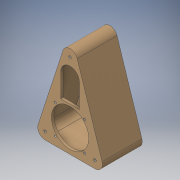
# Autodesk Inventor part: Nathan_New_LED_Speaker
Saved by Autodesk Inventor 2016 (Build 200138000, 138)
## iProperties
Created: 2018-09-25
Part Number: Nathan_New_LED_Speaker
Material: Generic
Document SubType Name: Modeling
Designer: Student
Density: 1 g/cm^3
Appearance: Default
Author: Student
Autodesk Inventor part; units mm, degrees
ref_plane "YZ Plane" through (0, 0, 0) normal (1, 0, 0) x (0, 1, 0)
ref_plane "XZ Plane" through (0, 0, 0) normal (0, 1, 0) x (-1, 0, 0)
ref_plane "XY Plane" through (0, 0, 0) normal (0, 0, 1) x (1, 0, 0)
sketch "Sketch1" plane through (0, 0, 0) normal (0, 0, 1) x (1, 0, 0)
  arc A0 (0.6195, 16.618) -> (12.7, 0) centre (12.7, 12.7) ccw
  arc A1 (63.5, 182.0332) -> (51.4195, 173.2512) centre (63.5, 169.3332) ccw
  line L0 (0.6195, 16.618) -> (51.4195, 173.2512)
  arc A2 (114.3, 0) -> (126.3805, 16.618) centre (114.3, 12.7) ccw
  arc A3 (75.5805, 173.2512) -> (63.5, 182.0332) centre (63.5, 169.3332) ccw
  line L1 (126.3805, 16.618) -> (75.5805, 173.2512)
  line L2 (12.7, 0) -> (114.3, 0)
  line L3 (63.5, 50.8) -> (63.5, 44.45)
  circle A4 centre (63.5, 44.45) radius 38.1
  circle A5 centre (33.655, 74.295) radius 2.1082
  circle A6 centre (93.345, 74.295) radius 2.1082
  circle A7 centre (93.345, 14.605) radius 2.1082
  circle A8 centre (33.655, 14.605) radius 2.1082
  line L4 (63.5, 82.55) -> (63.5, 86.36)
  line L5 (63.5, 86.36) -> (82.55, 86.36)
  line L6 (63.5, 86.36) -> (44.45, 86.36)
  line L7 (82.55, 86.36) -> (82.55, 134.62)
  line L8 (44.45, 86.36) -> (44.45, 134.62)
  arc A9 (82.55, 134.62) -> (44.45, 134.62) centre (63.5, 134.62) ccw
  point P0 (0, 0)
  dimension "d30" = 76.2
  dimension "d7" = 25.4
  dimension "d9" = 12.7
  dimension "d10" = 12.7
  dimension "d11" = 12.7
  dimension "d14" = 101.6
  dimension "d15" = 35.938
  dimension "d16" = 72.031
  dimension "d17" = 12.7
  dimension "d18" = 169.3332
  dimension "d19" = 109.3442
  dimension "d20" = 164.6651
  dimension "d21" = 164.6651
  dimension "d29" = 6.35
  dimension "d33" = 4.2164
  dimension "d34" = 4.2164
  dimension "d35" = 4.2164
  dimension "d36" = 4.2164
  dimension "d50" = 3.81
  dimension "d51" = 19.05
  dimension "d52" = 19.05
  dimension "d53" = 48.26
  dimension "d54" = 48.26
  constraints: 18 end point, 10 point on circle, 9 centre point, 4 vertical, 3 horizontal, 3 tangent, 1 coincident, 1 vertical alignment, 2 other
  measures "d7" diameter of A0
  measures "d9" radius of A2
  measures "d10" radius of A3
  measures "d11" radius of A1
  measures "d14" distance of L2.start L2.end
  measures "d15" angle of L1 L0
  measures "d16" angle of L2 L0
  measures "d17" distance from line of L2 A0.centre
  measures "d18" distance from line of L2 A1.centre
  measures "d19" distance from line of L1 A0.centre
  measures "d20" distance of L1.start L1.end
  measures "d21" distance of L0.start L0.end
  measures "d29" distance of L3.start L3.end
  measures "d33" diameter of A5
  measures "d34" diameter of A6
  measures "d35" diameter of A7
  measures "d36" diameter of A8
  measures "d50" distance of L4.start L4.end
  measures "d51" distance of L4.end L5.end
  measures "d52" distance of L4.end L6.end
  measures "d53" distance of L5.end L7.end
  measures "d54" distance of L6.end L8.end
extrude "Extrusion2" add sketch "Sketch1" along normal blind 5.08
sketch "Sketch2" plane through (0, 0, 0) normal (0, 0, -1) x (-1, 0, 0)
  line L0 (-126.3805, 16.618) -> (-75.5805, 173.2512) projected
  line L1 (-126.3805, 16.618) -> (-75.5805, 173.2512)
  line L2 (-51.4195, 173.2512) -> (-0.6195, 16.618) projected
  line L3 (-51.4195, 173.2512) -> (-0.6195, 16.618)
  line L4 (-12.7, 0) -> (-114.3, 0) projected
  line L5 (-114.3, 0) -> (-12.7, 0)
  arc A0 (-126.3805, 16.618) -> (-114.3, 0) centre (-114.3, 12.7) ccw projected
  arc A1 (-126.3805, 16.618) -> (-126.3805, 16.618) centre (-114.3, 12.7) ccw
  arc A2 (-12.7, 0) -> (-0.6195, 16.618) centre (-12.7, 12.7) ccw projected
  arc A3 (-12.7, 0) -> (-12.7, 0) centre (-12.7, 12.7) ccw
  arc A4 (-51.4195, 173.2512) -> (-75.5805, 173.2512) centre (-63.5, 169.3332) ccw projected
  arc A5 (-75.5805, 173.2512) -> (-75.5805, 173.2512) centre (-63.5, 169.3332) ccw
  arc A6 (-49.0034, 174.0348) -> (-77.9966, 174.0348) centre (-63.5, 169.3332) ccw
  arc A7 (-128.7966, 17.4016) -> (-114.3, -2.54) centre (-114.3, 12.7) ccw
  arc A8 (-12.7, -2.54) -> (1.7966, 17.4016) centre (-12.7, 12.7) ccw
  line L6 (-12.7, -2.54) -> (-114.3, -2.54)
  line L7 (-77.9966, 174.0348) -> (-128.7966, 17.4016)
  line L8 (-49.0034, 174.0348) -> (1.7966, 17.4016)
  point P0 (0, 0)
  dimension "d57" = 30.48
  dimension "d58" = 30.48
  dimension "d59" = 30.48
  constraints: 12 end point, 6 point on circle, 3 centre point, 3 coincident, 2 collinear, 2 horizontal, 1 tangent, 1 vertical alignment, 13 other
  measures "d57" diameter of A6
  measures "d58" diameter of A7
  measures "d59" diameter of A8
extrude "Extrusion3" add sketch "Sketch2" along normal blind 71.12 and the other way blind 5.08
sketch "Sketch3" plane through (0, 0, -71.12) normal (0, 0, -1) x (-1, 0, 0)
  line L0 (-12.7, -2.54) -> (-114.3, -2.54) projected
  line L1 (-114.3, -2.54) -> (-12.7, -2.54)
  line L2 (1.7966, 17.4016) -> (-49.0034, 174.0348) projected
  line L3 (1.7966, 17.4016) -> (-49.0034, 174.0348)
  line L4 (-128.7966, 17.4016) -> (-77.9966, 174.0348) projected
  line L5 (-77.9966, 174.0348) -> (-128.7966, 17.4016)
  arc A0 (-128.7966, 17.4016) -> (-114.3, -2.54) centre (-114.3, 12.7) ccw projected
  arc A1 (-128.7966, 17.4016) -> (-114.3, -2.54) centre (-114.3, 12.7) ccw
  arc A2 (-12.7, -2.54) -> (1.7966, 17.4016) centre (-12.7, 12.7) ccw projected
  arc A3 (-12.7, -2.54) -> (1.7966, 17.4016) centre (-12.7, 12.7) ccw
  arc A4 (-49.0034, 174.0348) -> (-77.9966, 174.0348) centre (-63.5, 169.3332) ccw
  point P0 (0, 0)
  constraints: 6 end point, 6 point on circle, 3 centre point, 2 collinear, 2 tangent, 1 horizontal
extrude "Extrusion4" add sketch "Sketch3" along normal blind 5.08
sketch "Sketch4" plane through (0, 0, -76.2) normal (0, 0, -1) x (-1, 0, 0)
  arc A0 (-49.0034, 174.0348) -> (-77.9966, 174.0348) centre (-63.5, 169.3332) ccw projected
  circle A1 centre (-63.5, 169.3332) radius 2.54
  arc A2 (-126.3805, 16.618) -> (-114.3, 0) centre (-114.3, 12.7) ccw projected
  circle A3 centre (-114.3, 12.7) radius 2.54
  arc A4 (-12.7, 0) -> (-0.6195, 16.618) centre (-12.7, 12.7) ccw projected
  circle A5 centre (-12.7, 12.7) radius 2.54
  point P0 (0, 0)
  dimension "d66" = 5.08
  dimension "d67" = 5.08
  dimension "d68" = 5.08
  constraints: 3 centre point, 3 coincident
  measures "d66" diameter of A1
  measures "d67" diameter of A3
  measures "d68" diameter of A5
extrude "Extrusion5" cut sketch "Sketch4" against normal blind 81.28
body "Solid2"
